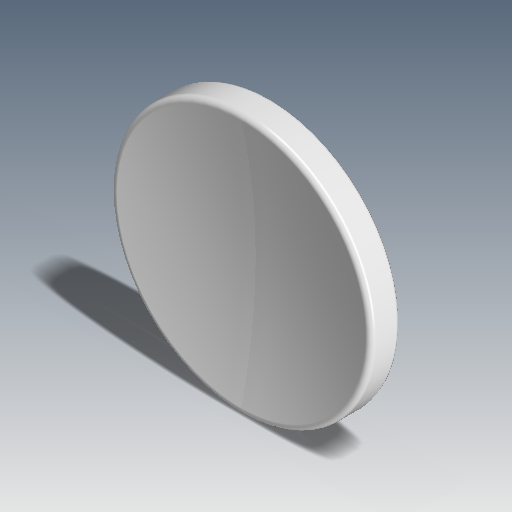
# Autodesk Inventor part: Plano Concanve Lens
Saved by Autodesk Inventor 2026 (Build 300175050, 175E)
## iProperties
Created: 2025-08-02
Part Number: Plano Concanve Lens
Material: Generic
Document SubType Name: Modeling
Designer: aman0
Density: 1 g/cm^3
Appearance: Default
Author: aman0
Autodesk Inventor part; units mm, degrees
ref_plane "YZ Plane" through (0, 0, 0) normal (1, 0, 0) x (0, 1, 0)
ref_plane "XZ Plane" through (0, 0, 0) normal (0, 1, 0) x (-1, 0, 0)
ref_plane "XY Plane" through (0, 0, 0) normal (0, 0, 1) x (1, 0, 0)
sketch "Sketch1" plane through (0, 0, 0) normal (0, 1, 0) x (-1, 0, 0)
  line L0 (12.5, 0) -> (12.5, 3)
  line L1 (12.5, 3) -> (-12.5, 3)
  line L2 (-12.5, 3) -> (-12.5, 0)
  line L3 (-12.5, 0) -> (12.5, 0)
  circle A0 centre (0, 53) radius 51.5388
  line L4 (0, 0) -> (0, 1.4612)
  point P0 (0, 0)
  point P1 (0, 3)
  dimension "d0" = 3
  dimension "d1" = 25
  dimension "d2" = 50
  constraints: 10 end point, 3 midpoint, 3 point on circle, 2 parallel, 2 vertical, 1 centre point, 1 horizontal alignment, 1 perpendicular, 1 vertical alignment
  measures "d0" distance of L0.start L0.end
  measures "d1" distance of L1.end L0.end
  measures "d2" distance of point (0, 3) A0.centre
revolve "Revolution1" add sketch "Sketch1" angle 360 about axis through (0, 0, 0) along (0, 0, 1) contours L3 L2 A0 L4
fillet "Fillet1" radius 0.5 2 edges at (-12.5, 0, 3) (-12.5, 0, 0)
body "Solid1"
